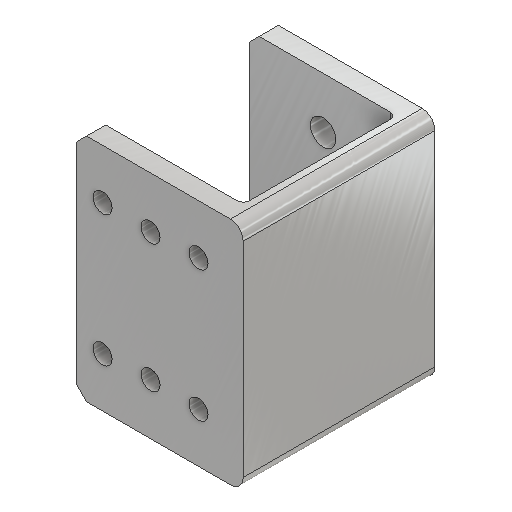
# Autodesk Inventor part: CNCM_ALU_Y_Axis_Belt_Mount_Bracket
Saved by Autodesk Inventor 2026.1 (Build 301233000, 233)
## iProperties
Created: 2016-03-27
Part Number: CNCM_ALU_Y_Axis_Belt_Mount_Bracket
Material: Ogólny
Document SubType Name: Modeling
Designer: Andrzej
Density: 1 g/cm^3
Appearance: Obrobione — aluminium
Mass: 8.15481 g
Surface Area: 60.6946 cm^2
Volume: 8.15481 cm^3
Author: Andrzej
Autodesk Inventor part; units mm, degrees
ref_plane "YZ Plane" through (0, 0, 0) normal (1, 0, 0) x (0, 1, 0)
ref_plane "XZ Plane" through (0, 0, 0) normal (0, 1, 0) x (-1, 0, 0)
ref_plane "XY Plane" through (0, 0, 0) normal (0, 0, 1) x (1, 0, 0)
sketch "Szkic1" plane through (0, 0, 0) normal (0, 0, 1) x (1, 0, 0)
  line L0 (-15.1556, -3.6171) -> (-15.1556, -6.6171)
  line L1 (-15.1556, -6.6171) -> (10.8444, -6.6171)
  line L2 (10.8444, -6.6171) -> (10.8444, 23.3829)
  line L3 (7.8444, 20.3829) -> (7.8444, -3.6171)
  line L4 (7.8444, -3.6171) -> (-15.1556, -3.6171)
  line L5 (-15.1556, 23.3829) -> (-15.1556, 20.3829)
  line L6 (-15.1556, 20.3829) -> (7.8444, 20.3829)
  line L7 (-15.1556, 23.3829) -> (10.8444, 23.3829)
  point P0 (0, 0)
  dimension "d1" = 26
  dimension "d2" = 30
  dimension "d87" = 3
  dimension "d88" = 24
  dimension "d89" = 3
  dimension "d90" = 3
  constraints: 16 end point, 4 perpendicular, 1 horizontal, 1 vertical
  measures "d1" distance of L0.end L1.end
  measures "d2" distance of L1.end L2.end
  measures "d87" distance of L5.start L5.end
  measures "d88" distance between parallel lines of L4 L6
  measures "d89" distance between parallel lines of L2 L3
  measures "d90" distance between parallel lines of L4 L1
extrude "Wyciągnięcie proste1" add sketch "Szkic1" along normal blind 36
fillet "Zaokrąglenie1" radius 1 2 edges at (7.8444, -3.6171, 18) (7.8444, 20.3829, 18)
chamfer "Faza4" distance 1.5 angle 45 4 edges at (-15.1556, -5.1171, 36) (-15.1556, -5.1171, 0) (-15.1556, 21.8829, 36) (-15.1556, 21.8829, 0)
fillet "Zaokrąglenie5" radius 2 2 edges at (10.8444, 8.3829, 36) (10.8444, 8.3829, 0)
sketch "Szkic7" plane through (-15.1556, -6.6171, 1.5) normal (0, -1, 0) x (1, 0, 0)
  arc A0 (24, -1.5) -> (26, 0.5) centre (24, 0.5) ccw projected
  line L0 (26, 0.5) -> (26, 32.5) projected
  arc A1 (26, 32.5) -> (24, 34.5) centre (24, 32.5) ccw projected
  line L1 (1.5, 34.5) -> (24, 34.5) projected
  line L2 (0, 33) -> (1.5, 34.5) projected
  line L3 (0, 0) -> (0, 33) projected
  line L4 (1.5, -1.5) -> (0, 0) projected
  line L5 (1.5, -1.5) -> (24, -1.5) projected
  line L6 (23, 34.5) -> (23, -1.5) projected
  point P0 (15.1556, -1.5)
  point P1 (19, 6.25)
  point P2 (4, 6.25)
  point P3 (4, 26.75)
  point P4 (19, 26.75)
  dimension "d95" = 4
  dimension "d96" = 4
  dimension "d97" = 4
  dimension "d98" = 4
  dimension "d99" = 7.75
  dimension "d100" = 7.75
  dimension "d101" = 7.75
  dimension "d102" = 7.75
  measures "d95" distance from line of L3 point (4, 6.25)
  measures "d96" distance from line of L3 point (4, 26.75)
  measures "d97" distance from line of L6 point (19, 6.25)
  measures "d98" distance from line of L6 point (19, 26.75)
  measures "d99" distance from line of L5 point (4, 6.25)
  measures "d100" distance from line of L5 point (19, 6.25)
  measures "d101" distance from line of L1 point (19, 26.75)
  measures "d102" distance from line of L1 point (4, 26.75)
hole "Otwór5" at (3.8444, -6.6171, 7.75) at (-11.1556, -6.6171, 7.75) at (-11.1556, -6.6171, 28.25) at (3.8444, -6.6171, 28.25) direction (0, 1, 0) diameter 3 depth 8 tip angle 118
sketch "Szkic8" plane through (-15.1556, 23.3829, 34.5) normal (0, 1, 0) x (1, 0, 0)
  arc A0 (26, 32.5) -> (24, 34.5) centre (24, 32.5) ccw projected
  line L0 (24, 34.5) -> (1.5, 34.5) projected
  line L1 (0, 33) -> (1.5, 34.5) projected
  line L2 (0, 33) -> (0, 0) projected
  line L3 (1.5, -1.5) -> (0, 0) projected
  line L4 (24, -1.5) -> (1.5, -1.5) projected
  arc A1 (24, -1.5) -> (26, 0.5) centre (24, 0.5) ccw projected
  line L5 (26, 32.5) -> (26, 0.5) projected
  line L6 (23, 34.5) -> (23, -1.5) projected
  point P0 (15.1556, 34.5)
  point P1 (11.5, 26.5)
  point P2 (11.5, 6.5)
  dimension "d110" = 11.5
  dimension "d111" = 23
  dimension "d112" = 11.5
  dimension "d113" = 20
  dimension "d114" = 36
  dimension "d115" = 8
  measures "d110" distance from line of L6 point (11.5, 26.5)
  measures "d111" distance between parallel lines of L2 L6
  measures "d112" distance from line of L6 point (11.5, 6.5)
  measures "d113" distance of point (11.5, 6.5) point (11.5, 26.5)
  measures "d114" distance between parallel lines of L4 L0
  measures "d115" distance from line of L0 point (11.5, 26.5)
hole "Otwór6" at (-3.6556, 23.3829, 8) at (-3.6556, 23.3829, 28) direction (0, -1, 0) diameter 4 depth 8 tip angle 118
sketch "Szkic9" plane through (-15.1556, -6.6171, 1.5) normal (0, -1, 0) x (1, 0, 0)
  circle A0 centre (11.5, 6.5) radius 2 projected
  circle A1 centre (11.5, 26.5) radius 2 projected
  circle A2 centre (11.5, 6.5) radius 1.5
  circle A3 centre (11.5, 26.5) radius 1.5
  point P0 (15.1556, -1.5)
  dimension "d123" = 3
  dimension "d124" = 3
  constraints: 2 centre point, 2 coincident
  measures "d123" diameter of A2
  measures "d124" diameter of A3
extrude "Wyciągnięcie proste4" cut sketch "Szkic9" against normal blind 10 contours A2 | A3
equation "\"d88\" = d2 - 2 * d87"
equation "\"d97\" = d95"
equation "\"d98\" = d96"
equation "\"d100\" = d99"
equation "\"d101\" = d99"
equation "\"d102\" = d99"
equation "\"d110\" = 0.5 * d111"
equation "\"d112\" = d110"
equation "\"d115\" = -0.5 * d113 + 0.5 * d114"
